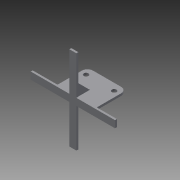
# Autodesk Inventor part: thrust-checker
Saved by Autodesk Inventor 2014 SP2 (Build 180247200, 247)
## iProperties
Created: 2018-11-23
Part Number: thrust-checker
Material: 一般
Document SubType Name: Modeling
Designer: hide
Density: 1 g/cm^3
Appearance: 既定
Author: hide
Autodesk Inventor part; units mm, degrees
ref_plane "YZ Plane" through (0, 0, 0) normal (1, 0, 0) x (0, 1, 0)
ref_plane "XZ Plane" through (0, 0, 0) normal (0, 1, 0) x (-1, 0, 0)
ref_plane "XY Plane" through (0, 0, 0) normal (0, 0, 1) x (1, 0, 0)
sketch "スケッチ1" plane through (0, 0, 0) normal (0, 0, 1) x (1, 0, 0)
  line L0 (-14, 0) -> (14, 0)
  line L1 (14, 0) -> (14, 23)
  line L2 (14, 23) -> (-14, 23)
  line L3 (-14, 23) -> (-14, 0)
  circle A0 centre (-10, 18) radius 1.65
  circle A1 centre (10, 18) radius 1.65
  point P0 (0, 0)
  dimension "d0" = 3.3
  dimension "d1" = 3.3
  dimension "d2" = 0
  dimension "d3" = 20
  dimension "d4" = 18
  dimension "d5" = 10
  dimension "d6" = 23
  dimension "d7" = 28
  dimension "d8" = 14
  dimension "d9" = 0
  constraints: 8 end point, 2 centre point, 2 parallel, 1 horizontal, 1 perpendicular
  measures "d0" diameter of A0
  measures "d1" diameter of A1
  measures "d2" vertical distance of A1.centre A0.centre
  measures "d3" distance of A0.centre A1.centre
  measures "d4" distance from line of L0 A0.centre
  measures "d5" horizontal distance of point (0, 0) A0.centre
  measures "d6" distance of L2.end L0.start
  measures "d7" distance between parallel lines of L1 L3
  measures "d8" distance from line of point (0, 0) L3
  measures "d9" distance from line of L0 point (0, 0)
extrude "押し出し1" add sketch "スケッチ1" along normal blind 1.6
sketch "スケッチ2" plane through (-14, 0, 0) normal (0, -1, 0) x (1, 0, 0)
  line L0 (0, 0) -> (28, 0) projected
  line L1 (28, 0) -> (28, 1.6) projected
  line L2 (0, 1.6) -> (28, 1.6) projected
  line L3 (0, 0) -> (0, 1.6) projected
  line L4 (-16, 3.25) -> (44, 3.25)
  line L5 (44, 3.25) -> (44, -1.75)
  line L6 (44, -1.75) -> (-16, -1.75)
  line L7 (-16, -1.75) -> (-16, 3.25)
  line L8 (11.5, 30.75) -> (16.5, 30.75)
  line L9 (16.5, 30.75) -> (16.5, -29.25)
  line L10 (16.5, -29.25) -> (11.5, -29.25)
  line L11 (11.5, -29.25) -> (11.5, 30.75)
  point P0 (14, 0)
  dimension "d12" = 60
  dimension "d13" = 60
  dimension "d14" = 5
  dimension "d15" = 5
  dimension "d16" = 1.75
  dimension "d17" = 2.5
  dimension "d18" = 30
  dimension "d19" = 29.25
  constraints: 16 end point, 4 parallel, 2 horizontal, 2 perpendicular
  measures "d12" distance between parallel lines of L10 L8
  measures "d13" distance between parallel lines of L7 L5
  measures "d14" distance between parallel lines of L11 L9
  measures "d15" distance between parallel lines of L6 L4
  measures "d16" distance between parallel lines of L0 L6
  measures "d17" distance from line of point (14, 0) L11
  measures "d18" distance from line of point (14, 0) L5
  measures "d19" distance between parallel lines of L10 L0
extrude "押し出し2" add sketch "スケッチ2" along normal blind 1.4
sketch "スケッチ3" plane through (0, 0, 0) normal (1, 0, 0) x (0, 1, 0)
  line L0 (-1.4, 3.25) -> (0, 3.25) projected
  line L1 (0, 30.75) -> (0, 3.25) projected
  line L2 (0, 30.75) -> (-1.4, 30.75) projected
  line L3 (-1.4, 3.25) -> (-1.4, 30.75) projected
  line L4 (0, -1.75) -> (-1.4, -1.75) projected
  line L5 (-1.4, -29.25) -> (-1.4, -1.75) projected
  line L6 (0, -29.25) -> (-1.4, -29.25) projected
  line L7 (0, -1.75) -> (0, -29.25) projected
  line L8 (0, 0) -> (23, 0) projected
  line L9 (23, 0) -> (23, 1.6) projected
  line L10 (0, 1.6) -> (23, 1.6) projected
  line L11 (0, 0) -> (0, 1.6) projected
  line L12 (0, 11.6) -> (10, 1.6)
  line L13 (10, 0) -> (0, -10)
  line L14 (10, 0) -> (10, 1.6)
  line L15 (0, 1.6) -> (10, 1.6)
  line L16 (10, 0) -> (0, 0)
  line L17 (0, -10) -> (0, 0)
  line L18 (0, 1.6) -> (0, 11.6)
  dimension "d22" = 45
  dimension "d23" = 45
  dimension "d24" = 0
  dimension "d25" = 10
  constraints: 14 end point, 4 point on line, 3 collinear, 2 perpendicular
  measures "d22" angle of L12 L10
  measures "d23" angle of L8 L13
  measures "d24" horizontal distance of L12.end L13.start
  measures "d25" distance from line of L10 L12.start
extrude "押し出し3" add sketch "スケッチ3" along normal mid plane 1.4 contours L1 L12 L10 L18
fillet "フィレット1" radius 4 2 edges at (-14, 23, 0.8) (14, 23, 0.8)
equation "\"d1\" = d0"
equation "\"d5\" = 0.5 * d3"
equation "\"d8\" = 0.5 * d7"
equation "\"d13\" = d12"
equation "\"d15\" = d14"
equation "\"d17\" = 0.5 * d15"
equation "\"d18\" = 0.5 * d13"
equation "\"d23\" = d22"
